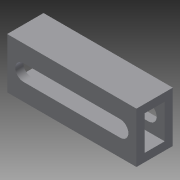
# Autodesk Inventor part: housing
Saved by Autodesk Inventor 2015 (Build 190159000, 159)
## iProperties
Created: 2015-04-06
Part Number: housing
Material: Generic
Document SubType Name: Modeling
Designer: WASHHSST
Density: 1 g/cm^3
Appearance: Default
Author: WASHHSST
Autodesk Inventor part; units mm, degrees
ref_plane "YZ Plane" through (0, 0, 0) normal (1, 0, 0) x (0, 1, 0)
ref_plane "XZ Plane" through (0, 0, 0) normal (0, 1, 0) x (-1, 0, 0)
ref_plane "XY Plane" through (0, 0, 0) normal (0, 0, 1) x (1, 0, 0)
sketch "Sketch1" plane through (0, 0, 0) normal (1, 0, 0) x (0, 1, 0)
  line L0 (0, 0) -> (26.9875, 0)
  line L1 (26.9875, 0) -> (26.9875, -15.875)
  line L2 (26.9875, -15.875) -> (0, -15.875)
  line L3 (0, -15.875) -> (0, 0)
  line L4 (33.3375, -22.225) -> (33.3375, 6.35)
  line L5 (33.3375, 6.35) -> (-6.35, 6.35)
  line L6 (-6.35, 6.35) -> (-6.35, -22.225)
  line L7 (-6.35, -22.225) -> (33.3375, -22.225)
  dimension "d0" = 26.9875
  dimension "d1" = 15.875
  dimension "d2" = 6.35
  constraints: 16 end point, 4 parallel, 2 perpendicular, 1 horizontal, 3 other
  measures "d0" distance of L1.end L2.end
  measures "d1" distance of L0.end L1.end
  measures "d2" distance between parallel lines of L1 L4
extrude "Extrusion1" add sketch "Sketch1" along normal blind 101.6
sketch "Sketch2" plane through (0, -6.35, 6.35) normal (0, 0, 1) x (1, 0, 0)
  line L0 (0, 39.6875) -> (0, 0) projected
  line L1 (0, 19.8437) -> (101.6, 19.8437)
  line L2 (101.6, 39.6875) -> (101.6, 0) projected
  circle A0 centre (12.7, 19.8437) radius 6.35
  line L3 (50.8, 39.6875) -> (50.8, 0)
  line L4 (0, 0) -> (101.6, 0) projected
  circle A1 centre (88.9, 19.8437) radius 6.35
  line L5 (88.9, 26.1937) -> (12.7, 26.1937)
  line L6 (12.7, 13.4937) -> (88.9, 13.4937)
  point P0 (0, 6.35)
  dimension "d5" = 12.7
  dimension "d6" = 12.7
  dimension "d7" = 50.8
  constraints: 8 end point, 4 point on circle, 3 midpoint, 2 centre point, 2 tangent, 1 horizontal, 1 point on line, 1 symmetric about line, 1 other
  measures "d5" diameter of A0
  measures "d6" distance from line of L0 A0.centre
  measures "d7" distance between parallel lines of L0 L3
extrude "Extrusion2" cut sketch "Sketch2" against normal through all contours A0 L1 | L1 A0 | A0 L5 L3 L1 | L1 L3 L6 A0 | L3 L1 A1 L6 | L3 L5 A1 L1 | A1 L1 | A1 L1
body "Solid1"
